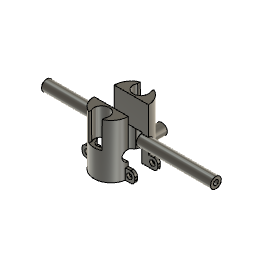
Badminton nozzle connector (Autodesk Fusion 360 design; units mm, degrees)
Autodesk Fusion 360 part; units mm, degrees
sketch "Sketch1" plane through (0, 0, 0) normal (0, 0, 1) x (1, 0, 0)
  circle A0 centre (0, 0) radius 7.65
  circle A1 centre (0, 0) radius 12.65
  dimension "d1" = 15.3
  dimension "d2" = 25.3
  constraint coincident A0.centre A1.centre
  measures "d1" diameter of A0
  measures "d2" diameter of A1
extrude "Extrude1" add sketch "Sketch1" along normal blind 20 makes body 1
ref_plane "WorkPlane1" through (0, 0, 20) normal (0, 0, 1) x (1, 0, 0)
ref_plane "WorkPlane2" through (0, 0, 40) normal (0, 0, 1) x (1, 0, 0)
sketch "Sketch4" plane through (0, 0, 40) normal (0, 0, 1) x (1, 0, 0)
  circle A0 centre (0, 0) radius 12.65
  circle A1 centre (0, 7) radius 5.65
  circle A2 centre (0, -7) radius 5.65
  line L0 (-5, -9) -> (5, -9)
  line L1 (5, -9) -> (5, -15)
  line L2 (5, -15) -> (-5, -15)
  line L3 (-5, -15) -> (-5, -9)
  line L4 (-5, 15) -> (5, 15)
  line L5 (-5, 9) -> (-5, 15)
  line L6 (5, 15) -> (5, 9)
  line L7 (5, 9) -> (-5, 9)
  dimension "d27" = 25.3
  dimension "d28" = 11.3
  dimension "d29" = 11.3
  dimension "d30" = 10
  dimension "d31" = 6
  dimension "d32" = 10
  dimension "d33" = 6
  constraint coincident A0.centre origin
  constraint horizontal L0
  constraint vertical L1
  constraint horizontal L2
  constraint vertical L3
  constraint horizontal L4
  constraint vertical L6
  constraint horizontal L7
  constraint vertical L5
  measures "d27" diameter of A0
  measures "d28" diameter of A1
  measures "d29" diameter of A2
  measures "d30" distance of L0.start L0.end
  measures "d31" distance of L0.start L2.end
  measures "d32" distance of L4.start L4.end
  measures "d33" distance of L5.start L4.start
extrude "Extrude4" add sketch "Sketch4" against normal blind 20 contours A0 A1 A2 L1 L3 L5 L6 | A0 A1 L6 | A0 A2 L1 | A0 A1 L5 | A1 L5 L6 L7 | A1 L5 L6 L7 | A0 A2 L3 | A2 L0 L1 L3 | A2 L0 L1 L3 bodies 1
extrude "Extrude5" cut sketch "Sketch4" against normal blind 20 draft -0.5 contours A0 A1 L6 | A0 L4 L5 L6 | A0 L1 L2 L3 | A0 A2 L1 | A0 A1 L5 | A1 L5 L6 L7 | A1 L5 L6 L7 | A0 A2 L3 | A2 L0 L1 L3 | A2 L0 L1 L3 bodies 1
sketch "Sketch3" plane through (0, 0, 0) normal (0, 1, 0) x (1, 0, 0)
  line L0 (11.5, -8) -> (19.5, -8)
  line L1 (19.5, -8) -> (19.5, 0)
  line L2 (19.5, 0) -> (11.5, 0)
  line L3 (11.5, 0) -> (11.5, -8)
  circle A0 centre (15.5, -4) radius 2
  circle A1 centre (-15.5, -4) radius 2
  line L4 (-19.5, -8) -> (-11.5, -8)
  line L5 (-11.5, -8) -> (-11.5, 0)
  line L6 (-11.5, 0) -> (-19.5, 0)
  line L7 (-19.5, 0) -> (-19.5, -8)
  dimension "d16" = 8
  dimension "d17" = 8
  dimension "d18" = 4
  dimension "d19" = 8
  dimension "d20" = 8
  dimension "d21" = 4
  constraint horizontal L0
  constraint vertical L1
  constraint horizontal L2
  constraint vertical L3
  constraint horizontal L4
  constraint vertical L5
  constraint horizontal L6
  constraint vertical L7
  measures "d16" distance of L0.start L0.end
  measures "d17" distance of L0.start L2.end
  measures "d18" diameter of A0
  measures "d19" distance of L4.end L4.start
  measures "d20" distance of L6.end L4.start
  measures "d21" diameter of A1
extrude "Extrude3" add sketch "Sketch3" along normal blind 2 and the other way blind 2 bodies 1
sketch "Sketch5" plane through (0, 0, 20) normal (0, 0, 1) x (-1, 0, 0)
  arc A0 (4.8255, 11.6935) -> (-4.8255, 11.6935) centre (0, 0) ccw
  line L0 (-4.8255, 11.6935) -> (-4.8255, 9.5876)
  arc A1 (-4.8255, 9.5876) -> (-5.2769, 5.5387) centre (0, 7) ccw
  arc A2 (5.2769, 5.5387) -> (-5.2769, 5.5387) centre (0, 0) ccw
  arc A3 (5.2769, 5.5387) -> (4.8255, 9.5876) centre (0, 7) ccw
  line L1 (4.8255, 9.5876) -> (4.8255, 11.6935)
  circle A4 centre (0, 7) radius 3.5
  circle A5 centre (0, -7) radius 3.5
  dimension "d39" = 7
  dimension "d40" = 7
  constraint concentric A1 A4
  measures "d39" diameter of A4
  measures "d40" diameter of A5
extrude "Extrude6" cut sketch "Sketch5" against normal blind 20 contours A2 A4 | A2 A4 | A5 bodies 1
sketch "Sketch7" plane through (0, 0, 0) normal (0, 0, 1) x (1, 0, 0)
  line L0 (0, 0) -> (40, 0)
  line L1 (40, 0) -> (40, -9)
  line L2 (40, -9) -> (0, -9)
  line L3 (0, -9) -> (0, 0)
  dimension "d48" = 40
  constraint horizontal L0
  constraint vertical L1
  constraint horizontal L2
  constraint vertical L3
  constraint coincident L0.start L3.end
  measures "d48" distance of L0.start L0.end
ref_plane "WorkPlane7" through (12.65, 0, 40) normal (0.825484, 0, 0.564425) x (0, 1, 0)
sketch "Sketch11" plane through (0, 0, 0) normal (0, 0, 1) x (1, 0, 0)
  line L0 (-10, -10) -> (10, -10)
  line L1 (10, -10) -> (10, 10)
  line L2 (10, 10) -> (-10, 10)
  line L3 (-10, 10) -> (-10, -10)
  constraint horizontal L0
  constraint vertical L1
  constraint horizontal L2
  constraint vertical L3
ref_plane "WorkPlane11" through (12.65, 0, 0) normal (1, 0, 0) x (0, 1, 0)
sketch "Sketch14" plane through (12.65, 0, 0) normal (1, 0, 0) x (0, 1, 0)
  circle A0 centre (0, 15) radius 4
  dimension "d72" = 8
  measures "d72" diameter of A0
extrude "Extrude12" add sketch "Sketch14" along normal blind 50 and the other way blind 5 separate body makes body 2
sketch "Sketch15" plane through (62.65, 0, 0) normal (1, 0, 0) x (0, 1, 0)
  circle A0 centre (0, 15) radius 4
  circle A1 centre (0, 15) radius 1.8
  dimension "d77" = 3.6
  constraint concentric A0 A1
  measures "d77" diameter of A1
extrude "Extrude13" cut sketch "Sketch15" against normal blind 15 contours A1 bodies 1 2
mirror "Mirror2" about plane through (0, 0, 0) normal (1, 0, 0) of bodies 2 makes body 3
ref_plane "WorkPlane12" through (0, 12.65, 0) normal (0, 1, 0) x (0, 0, 1)
sketch "Sketch16" plane through (0, 12.65, 0) normal (0, 1, 0) x (1, 0, 0)
  circle A0 centre (0, -7) radius 4
  dimension "d83" = 8
  measures "d83" diameter of A0
extrude "Extrude14" add sketch "Sketch16" along normal blind 10 and the other way blind 2 bodies 1
sketch "Sketch17" plane through (0, 22.65, 0) normal (0, 1, 0) x (-1, 0, 0)
  circle A0 centre (0, 7) radius 4
  circle A1 centre (0, 7) radius 1.8
  dimension "d88" = 3.6
  constraint concentric A0 A1
  measures "d88" diameter of A1
extrude "Extrude15" cut sketch "Sketch17" against normal blind 8 contours A1 bodies 1
split "Split1" by plane through (0, 0, 0) normal (0, 1, 0) bodies 1 makes body 4 at (-6.936, 10.579, 13.3333)
move_body "Move1" bodies 1 to x (1, 0, 0) y (0, 1, 0) z (0, 0, 1) at (0, -15, 0)
sketch "Sketch18" plane through (12.65, 0, 0) normal (1, 0, 0) x (0, 1, 0)
  circle A0 centre (-15, 15) radius 4
  dimension "d91" = 8
  measures "d91" diameter of A0
extrude "Extrude16" cut sketch "Sketch18" against normal blind 26 bodies 1
fillet "Fillet1" radius 3 8 edges at (-19.5, -16, 8) (-19.5, -16, 0) (19.5, -16, 8) (19.5, -16, 0) (-19.5, 1, 8) (-19.5, 1, 0) (19.5, 1, 0) (19.5, 1, 8) on bodies 1 4
combine "Combine1" operation add target body 2 tool bodies 4 3
